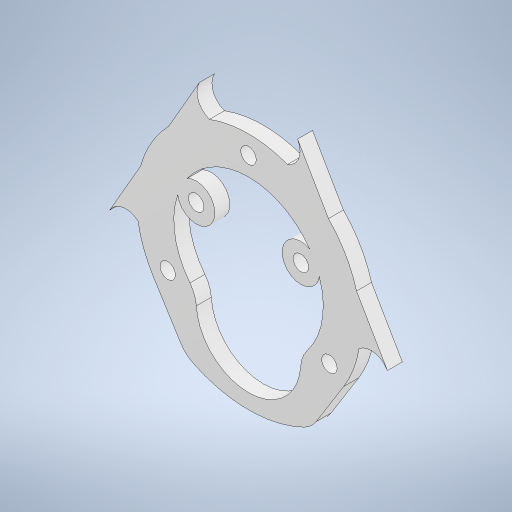
# Autodesk Inventor part: Support Ring
Saved by Autodesk Inventor 2023.2 (Build 272271000, 271)
## iProperties
Created: 2023-06-11
Part Number: Support Ring
Material: UHMW, White
Document SubType Name: Modeling
Designer: Nathan Cai
Mass: 19.9722 g
Surface Area: 139.915 cm^2
Volume: 21.247 cm^3
Density: 0.94 g/cm^3
Appearance: Smooth - White
Author: Nathan Cai
Autodesk Inventor part; units mm, degrees
ref_plane "YZ Plane" through (0, 0, 0) normal (1, 0, 0) x (0, 1, 0)
ref_plane "XZ Plane" through (0, 0, 0) normal (0, 1, 0) x (-1, 0, 0)
ref_plane "XY Plane" through (0, 0, 0) normal (0, 0, 1) x (1, 0, 0)
sketch "Sketch1" plane through (0, 0, 0) normal (0, 0, 1) x (1, 0, 0)
  circle A0 centre (0, 0) radius 47.625
  line L0 (0, 0) -> (0, 47.625) construction
  circle A1 centre (0, 39.6875) radius 7.9375 construction
  circle A2 centre (0, 39.6875) radius 3.302
  circle A3 centre (-34.3704, -19.8437) radius 3.302
  circle A4 centre (34.3704, -19.8438) radius 3.302
  circle A5 centre (0, 0) radius 31.75
  circle A6 centre (0, -25.4) radius 22.225 construction
  circle A7 centre (0, -25.4) radius 22.225
  circle A8 centre (0, 0) radius 53.975
  line L1 (0, 0) -> (-26.9875, -46.7437)
  line L2 (0, 0) -> (26.9875, -46.7437)
  line L3 (-26.9875, -46.7437) -> (-40.4202, -25.1863)
  line L4 (26.9875, -46.7437) -> (40.4202, -25.1863)
  circle A9 centre (-34.3704, -19.8437) radius 7.9375 construction
  circle A10 centre (34.3704, -19.8438) radius 7.9375 construction
  circle A11 centre (0, 39.6875) radius 4.7625 construction
  circle A12 centre (-34.3704, -19.8437) radius 4.7625 construction
  circle A13 centre (34.3704, -19.8438) radius 4.7625 construction
  circle A14 centre (22.225, 11.2503) radius 20.6375 construction
  circle A15 centre (22.225, 11.2503) radius 3.302
  circle A16 centre (22.225, 11.2503) radius 7.9375
  circle A17 centre (-22.225, 11.2503) radius 3.302
  circle A18 centre (-22.225, 11.2503) radius 7.9375
  point P0 (-22.0748, -22.8203)
  point P1 (22.0748, -22.8203)
  point P2 (26.9875, -46.7437)
  point P3 (40.4202, -25.1863)
  dimension "d12" = 107.95
  dimension "d0" = 95.25
  dimension "d1" = 15.875
  dimension "d2" = 6.604
  dimension "d5" = 360
  dimension "d7" = 63.5
  dimension "d10" = 44.45
  dimension "d11" = 44.45
  dimension "d13" = 30
  dimension "d17" = 360
  dimension "d21" = 9.525
  dimension "d24" = 360
  dimension "d61" = 41.275
  dimension "d62" = 22.225
  dimension "d63" = 6.604
  dimension "d64" = 15.875
  constraints: 18 centre point, 10 end point, 9 coincident, 4 symmetric about line, 4 tangent, 2 point on circle, 2 point on line, 1 vertical, 26 other
  measures "d0" diameter of A0
  measures "d1" diameter of A1
  measures "d2" diameter of A2
  measures "d7" diameter of A5
  measures "d10" diameter of A6
  measures "d11" diameter of A7
  measures "d13" angle of L0 L1
  measures "d21" diameter of A11
  measures "d61" diameter of A14
  measures "d62" distance from line of L0 A14.centre
  measures "d63" diameter of A15
  measures "d64" diameter of A16
extrude "Extrusion1" add sketch "Sketch1" along normal blind 6.35 contours A0 L2 A7 A5 A16 A18 L1 | A0 L1 L3 | L4 L2 A0 | L1 A7 A0 | A0 L2 A8 L1 | A0 A7 L2 | A18 A5 | A5 A18 | A16 A5 | A5 A16
fillet "Fillet1" radius 12.7 4 edges at (-22.0748, -22.8203, 3.175) (22.0748, -22.8203, 3.175) (26.9875, -46.7437, 3.175) (-26.9875, -46.7437, 3.175)
sketch "Sketch2" plane through (0, 0, 0) normal (0, 0, -1) x (-1, 0, 0)
  point P0 (-38.1661, -38.1661)
  point P1 (-52.1358, -13.9698)
  point P2 (-13.9698, 52.1358)
  point P3 (13.9698, 52.1358)
  point P4 (52.1358, -13.9698)
  point P5 (38.1661, -38.1661)
hole "Hole1" at (38.1661, -38.1661, 0) at (52.1358, -13.9698, 0) at (13.9698, 52.1358, 0) at (-13.9698, 52.1358, 0) at (-52.1358, -13.9698, 0) at (-38.1661, -38.1661, 0) direction (0, 0, 1) diameter 6.604 end through all
sketch "Sketch3" plane through (0, 0, 0) normal (0, 0, -1) x (-1, 0, 0)
  circle A0 centre (13.9698, 52.1358) radius 3.302 projected
  circle A1 centre (13.9698, 52.1358) radius 7.9375
  circle A2 centre (-13.9698, 52.1358) radius 3.302 projected
  circle A3 centre (-13.9698, 52.1358) radius 7.9375
  circle A4 centre (-52.1358, -13.9698) radius 7.9375
  circle A5 centre (-38.1661, -38.1661) radius 7.9375
  circle A6 centre (38.1661, -38.1661) radius 7.9375
  circle A7 centre (52.1358, -13.9698) radius 7.9375
  line L0 (20.8438, 56.1046) -> (59.0099, -10.001)
  line L1 (-59.0099, -10.001) -> (-20.8438, 56.1046)
  line L2 (38.1661, -46.1036) -> (-38.1661, -46.1036)
  arc A8 (44.3097, -15.2947) -> (8.9093, 46.0207) centre (-55.8649, -32.2536) ccw
  arc A9 (-8.9093, 46.0207) -> (-44.3097, -15.2947) centre (55.8649, -32.2536) ccw
  arc A10 (-35.4004, -30.726) -> (35.4004, -30.726) centre (0, 64.5072) ccw
  circle A11 centre (0, 0) radius 61.9125
  circle A12 centre (0, 39.6875) radius 3.302 projected
  circle A13 centre (0, 39.6875) radius 7.9375
  circle A14 centre (0, 0) radius 39.6875 construction
  point P0 (-44.3097, -15.2947)
  point P1 (-8.9093, 46.0207)
  point P2 (-16.0241, 59.8029)
  point P3 (-59.8029, -16.0241)
  point P4 (59.8029, -16.0241)
  point P5 (16.0241, 59.8029)
  dimension "d33" = 15.875
  dimension "d34" = 15.875
  dimension "d37" = 360
  dimension "d41" = 360
  dimension "d43" = 101.6
  dimension "d46" = 360
  dimension "d50" = 15.875
  constraints: 11 centre point, 10 point on circle, 6 end point, 5 coincident, 5 tangent, 1 vertical alignment, 38 other
  measures "d33" diameter of A1
  measures "d34" diameter of A3
  measures "d43" radius of A8
  measures "d50" diameter of A13
extrude "Extrusion2" add sketch "Sketch3" against normal blind 6.35 contours A1 L0 A7 A8 | A3 A9 A4 L1
sketch "Sketch4" plane through (0, 0, 6.35) normal (0, 0, 1) x (1, 0, 0)
  arc A0 (-46.9558, -7.9555) -> (-40.4202, -25.1863) centre (0, 0) ccw projected
  line L0 (-40.4202, -25.1863) -> (-28.7871, -43.8556) projected
  arc A1 (-28.7871, -43.8556) -> (-23.5495, -48.5667) centre (-18.0084, -37.1392) ccw projected
  arc A2 (-23.5495, -48.5667) -> (23.5495, -48.5667) centre (0, 0) ccw projected
  arc A3 (23.5495, -48.5667) -> (28.7871, -43.8556) centre (18.0084, -37.1392) ccw projected
  line L1 (28.7871, -43.8556) -> (40.4202, -25.1863) projected
  arc A4 (40.4202, -25.1863) -> (46.9558, -7.9555) centre (0, 0) ccw projected
  line L2 (59.0099, -10.001) -> (20.8438, 56.1046) projected
  arc A5 (16.5883, 44.6427) -> (-16.5883, 44.6427) centre (0, 0) ccw projected
  line L3 (-20.8438, 56.1046) -> (-59.0099, -10.001) projected
  arc A6 (16.6623, -41.2089) -> (42.2431, -13.832) centre (0, 0) ccw projected
  arc A7 (16.6623, -41.2089) -> (13.6328, -42.9527) centre (21.423, -52.9828) ccw projected
  arc A8 (-13.6328, -42.9527) -> (13.6328, -42.9527) centre (0, -25.4) ccw projected
  arc A9 (-13.6328, -42.9527) -> (-16.6623, -41.2089) centre (-21.423, -52.9828) ccw projected
  arc A10 (-42.2431, -13.832) -> (-16.6623, -41.2089) centre (0, 0) ccw projected
  arc A11 (-42.4649, -6.6838) -> (-42.2431, -13.832) centre (-30.1736, -9.88) ccw projected
  arc A12 (-15.4441, 40.1175) -> (-42.4649, -6.6838) centre (55.8649, -32.2536) ccw projected
  arc A13 (-9.1427, 43.4996) -> (-15.4441, 40.1175) centre (-6.5305, 31.0711) ccw projected
  arc A14 (9.1427, 43.4996) -> (-9.1427, 43.4996) centre (0, 0) ccw projected
  arc A15 (15.4441, 40.1175) -> (9.1427, 43.4996) centre (6.5305, 31.0711) ccw projected
  arc A16 (42.4649, -6.6838) -> (15.4441, 40.1175) centre (-55.8649, -32.2536) ccw projected
  arc A17 (42.2431, -13.832) -> (42.4649, -6.6838) centre (30.1736, -9.88) ccw projected
  arc A18 (17.6725, 42.3791) -> (9.7957, 46.6067) centre (6.5305, 31.0711) ccw
  arc A19 (9.7957, 46.6067) -> (-9.7957, 46.6067) centre (0, 0) ccw
  arc A20 (-9.7957, 46.6067) -> (-17.6725, 42.3791) centre (-6.5305, 31.0711) ccw
  arc A21 (-17.6725, 42.3791) -> (-45.5377, -5.8847) centre (55.8649, -32.2536) ccw
  arc A22 (-45.5377, -5.8847) -> (-45.2604, -14.82) centre (-30.1736, -9.88) ccw
  arc A23 (-45.2604, -14.82) -> (-17.8525, -44.1523) centre (0, 0) ccw
  arc A24 (-15.5803, -45.4602) -> (-17.8525, -44.1523) centre (-21.423, -52.9828) ccw
  arc A25 (-15.5803, -45.4602) -> (15.5803, -45.4602) centre (0, -25.4) ccw
  arc A26 (17.8525, -44.1523) -> (15.5803, -45.4602) centre (21.423, -52.9828) ccw
  arc A27 (17.8525, -44.1523) -> (45.2604, -14.82) centre (0, 0) ccw
  arc A28 (45.2604, -14.82) -> (45.5377, -5.8847) centre (30.1736, -9.88) ccw
  arc A29 (45.5377, -5.8847) -> (17.6725, 42.3791) centre (-55.8649, -32.2536) ccw
  circle A30 centre (52.1358, -13.9698) radius 7.9375
  circle A31 centre (38.1661, -38.1661) radius 7.9375
  line L4 (0, 0) -> (0, -47.625) construction
  arc A32 (-13.6328, -42.9527) -> (13.6328, -42.9527) centre (0, -25.4) ccw projected
  circle A33 centre (13.9698, 52.1358) radius 3.302 projected
  circle A34 centre (13.9698, 52.1358) radius 7.9375
  circle A35 centre (-52.1358, -13.9698) radius 7.9375
  circle A36 centre (-38.1661, -38.1661) radius 7.9375
  circle A37 centre (-13.9698, 52.1358) radius 7.9375
  circle A38 centre (22.225, 11.2503) radius 7.9375 projected
  circle A39 centre (-22.225, 11.2503) radius 7.9375 projected
  arc A40 (16.5883, 44.6427) -> (20.8438, 56.1046) centre (13.9698, 52.1358) ccw projected
  arc A41 (-20.8438, 56.1046) -> (-16.5883, 44.6427) centre (-13.9698, 52.1358) ccw projected
  arc A42 (-46.9558, -7.9555) -> (-59.0099, -10.001) centre (-52.1358, -13.9698) ccw projected
  arc A43 (59.0099, -10.001) -> (46.9558, -7.9555) centre (52.1358, -13.9698) ccw projected
  point P0 (-46.019, -8.9112)
  point P1 (-15.2922, 44.3093)
  point P2 (15.2922, 44.3093)
  point P3 (46.019, -8.9112)
  point P4 (37.2448, -30.2822)
  point P5 (30.5492, -40.3992)
  point P6 (-30.5492, -40.3992)
  point P7 (-30.683, -40.8131)
  point P8 (-44.6427, -16.5883)
  point P9 (9.7957, 46.6067)
  point P10 (-7.9555, 46.9558)
  point P11 (-16.5883, 44.6427)
  point P12 (-9.7957, 46.6067)
  point P13 (-44.7415, -16.8555)
  point P14 (-46.9558, -7.9555)
  point P15 (44.6427, -16.5883)
  point P16 (7.9555, 46.9558)
  point P17 (46.9558, -7.9555)
  point P18 (16.5883, 44.6427)
  point P19 (36.6872, -30.3676)
  point P20 (30.3676, -36.6872)
  point P21 (-30.3676, -36.6872)
  point P22 (-36.6872, -30.3676)
  point P23 (45.2604, -14.82)
  point P24 (-44.6427, -16.5883)
  point P25 (-40.4202, -25.1863)
  point P26 (-40.4202, -25.1863)
  point P27 (44.6427, -16.5883)
  point P28 (-37.2448, -30.2822)
  point P29 (30.683, -40.8131)
  dimension "d54" = 3.175
  dimension "d55" = 15.875
  dimension "d56" = 15.875
  dimension "d57" = 15.875
  constraints: 26 point on circle, 18 centre point, 3 symmetric about line, 2 end point, 1 coincident, 14 other
  measures "d54" radial gap between concentric circles of A16 A29
  measures "d55" diameter of A30
  measures "d56" diameter of A31
  measures "d57" diameter of A34
sketch "Sketch5" plane through (0, 0, 6.35) normal (0, 0, 1) x (1, 0, 0)
  arc A0 (-27.9283, -37.7947) -> (27.9283, -37.7947) centre (0, -31.75) ccw projected
  line L0 (0, 0) -> (0, -31.75) construction
  circle A1 centre (0, -60.325) radius 6.35
  dimension "d65" = 12.7
  constraints: 2 end point, 1 centre point, 1 point on circle, 1 vertical
  measures "d65" diameter of A1
equation "\"d0\" = Ring_ID"
equation "\"d10\" = Pulley_OD"
equation "\"d11\" = Pulley_OD"
equation "\"d61\" = Brass_OD"
equation "\"d62\" = Brass_Offset"
equation "\"Ring_ID\" = 95.25"
equation "\"Pulley_OD\" = 44.45"
equation "\"Brass_OD\" = 41.275"
equation "\"Brass_Offset\" = 22.225"
body "Solid1"
